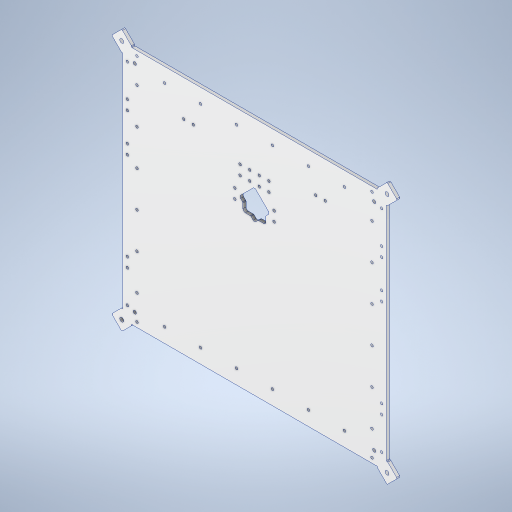
# Autodesk Inventor part: Printer Base Plate RevII
Saved by Autodesk Inventor 2024 (Build 280153000, 153)
## iProperties
Created: 2024-10-26
Part Number: Printer Base Plate RevII
Material: Aluminum 6061
Document SubType Name: Modeling
Designer: Ishaan
Density: 2.7 g/cm^3
Appearance: Aluminum - Flat
Author: Ishaan
Autodesk Inventor part; units mm, degrees
ref_plane "YZ Plane" through (0, 0, 0) normal (1, 0, 0) x (0, 1, 0)
ref_plane "XZ Plane" through (0, 0, 0) normal (0, 1, 0) x (-1, 0, 0)
ref_plane "XY Plane" through (0, 0, 0) normal (0, 0, 1) x (1, 0, 0)
sketch "Sketch1" plane through (0, 0, 0) normal (0, 0, 1) x (1, 0, 0)
  line L0 (275, -250) -> (-275, -250)
  line L1 (-275, -250) -> (-275, 250)
  line L2 (-275, 250) -> (275, 250)
  line L3 (275, 250) -> (275, -250)
  line L4 (275, -250) -> (-275, 250) construction
  line L5 (-275, -250) -> (275, 250) construction
  point P0 (0, 0)
  dimension "d0" = 550
  dimension "d1" = 500
  constraints: 12 end point, 2 midpoint, 2 parallel, 1 horizontal, 1 perpendicular
  measures "d0" distance of L1.end L2.end
  measures "d1" distance of L0.end L1.end
extrude "Extrusion1" add sketch "Sketch1" against normal blind 6.35
sketch "Sketch2" plane through (0, 0, 0) normal (0, 0, 1) x (1, 0, 0)
  line L0 (-235, 210) -> (-275, 210) construction
  line L1 (-275, 210) -> (-275, 250) construction
  line L2 (-275, 250) -> (-235, 250) construction
  line L3 (-235, 250) -> (-235, 210) construction
  line L4 (-235, 210) -> (-275, 250) construction
  line L5 (-275, 210) -> (-235, 250) construction
  line L6 (275, 210) -> (235, 210) construction
  line L7 (235, 210) -> (235, 250) construction
  line L8 (235, 250) -> (275, 250) construction
  line L9 (275, 250) -> (275, 210) construction
  line L10 (275, 210) -> (235, 250) construction
  line L11 (235, 210) -> (275, 250) construction
  line L12 (40, 122) -> (-40, 122) construction
  line L13 (-40, 122) -> (-40, 162) construction
  line L14 (-40, 162) -> (40, 162) construction
  line L15 (40, 162) -> (40, 122) construction
  line L16 (40, 122) -> (-40, 162) construction
  line L17 (-40, 122) -> (40, 162) construction
  line L18 (-235, -250) -> (-275, -250) construction
  line L19 (-275, -250) -> (-275, -210) construction
  line L20 (-275, -210) -> (-235, -210) construction
  line L21 (-235, -210) -> (-235, -250) construction
  line L22 (-235, -250) -> (-275, -210) construction
  line L23 (-275, -250) -> (-235, -210) construction
  line L24 (-275, 250) -> (-275, -250) construction
  line L25 (-275, -250) -> (275, -250) construction
  line L26 (275, -250) -> (235, -250) construction
  line L27 (235, -250) -> (235, -210) construction
  line L28 (235, -210) -> (275, -210) construction
  line L29 (275, -210) -> (275, -250) construction
  line L30 (275, -250) -> (235, -210) construction
  line L31 (235, -250) -> (275, -210) construction
  line L32 (275, -250) -> (275, 250) construction
  line L33 (-255, 122) -> (-275, 122) construction
  line L34 (-275, 122) -> (-275, 162) construction
  line L35 (-275, 162) -> (-255, 162) construction
  line L36 (-255, 162) -> (-255, 122) construction
  line L37 (-255, 122) -> (-275, 162) construction
  line L38 (-275, 122) -> (-255, 162) construction
  line L39 (275, 122) -> (255, 122) construction
  line L40 (255, 122) -> (255, 162) construction
  line L41 (255, 162) -> (275, 162) construction
  line L42 (275, 162) -> (275, 122) construction
  line L43 (275, 122) -> (255, 162) construction
  line L44 (255, 122) -> (275, 162) construction
  line L45 (-117.5, 165) -> (-157.5, 165) construction
  line L46 (-157.5, 165) -> (-157.5, 185) construction
  line L47 (-157.5, 185) -> (-117.5, 185) construction
  line L48 (-117.5, 185) -> (-117.5, 165) construction
  line L49 (-117.5, 165) -> (-157.5, 185) construction
  line L50 (-157.5, 165) -> (-117.5, 185) construction
  line L51 (157.5, 165) -> (117.5, 165) construction
  line L52 (117.5, 165) -> (117.5, 185) construction
  line L53 (117.5, 185) -> (157.5, 185) construction
  line L54 (157.5, 185) -> (157.5, 165) construction
  line L55 (157.5, 165) -> (117.5, 185) construction
  line L56 (117.5, 165) -> (157.5, 185) construction
  line L57 (-137.5, 175) -> (137.5, 175) construction
  line L58 (-255, -162) -> (-275, -162) construction
  line L59 (-275, -162) -> (-275, -122) construction
  line L60 (-275, -122) -> (-255, -122) construction
  line L61 (-255, -122) -> (-255, -162) construction
  line L62 (-255, -162) -> (-275, -122) construction
  line L63 (-275, -162) -> (-255, -122) construction
  line L64 (-255, 42) -> (-275, 42) construction
  line L65 (-275, 42) -> (-275, 82) construction
  line L66 (-275, 82) -> (-255, 82) construction
  line L67 (-255, 82) -> (-255, 42) construction
  line L68 (-255, 42) -> (-275, 82) construction
  line L69 (-275, 42) -> (-255, 82) construction
  line L70 (275, 42) -> (255, 42) construction
  line L71 (255, 42) -> (255, 82) construction
  line L72 (255, 82) -> (275, 82) construction
  line L73 (275, 82) -> (275, 42) construction
  line L74 (275, 42) -> (255, 82) construction
  line L75 (255, 42) -> (275, 82) construction
  line L76 (275, -162) -> (255, -162) construction
  line L77 (255, -162) -> (255, -122) construction
  line L78 (255, -122) -> (275, -122) construction
  line L79 (275, -122) -> (275, -162) construction
  line L80 (275, -162) -> (255, -122) construction
  line L81 (255, -162) -> (275, -122) construction
  line L82 (-275, 220) -> (-235, 220) construction
  line L83 (-275, -250) -> (-275, 250) construction
  line L84 (-275, 132) -> (-255, 132) construction
  line L85 (-275, -220) -> (-235, -220) construction
  line L86 (-275, -132) -> (-255, -132) construction
  line L87 (-255, 42) -> (-255, -122) construction
  line L88 (-255, -40) -> (0, -40) construction
  line L89 (0, 122) -> (0, -250) construction
  line L90 (-245, 220) -> (-265, 220) construction
  line L91 (-265, 220) -> (-265, 240) construction
  line L92 (-265, 240) -> (-245, 240) construction
  line L93 (-245, 240) -> (-245, 220) construction
  line L94 (-245, 220) -> (-265, 240) construction
  line L95 (-265, 220) -> (-245, 240) construction
  line L96 (265, 220) -> (245, 220) construction
  line L97 (245, 220) -> (245, 240) construction
  line L98 (245, 240) -> (265, 240) construction
  line L99 (265, 240) -> (265, 220) construction
  line L100 (265, 220) -> (245, 240) construction
  line L101 (245, 220) -> (265, 240) construction
  line L102 (265, 152) -> (265, 132) construction
  line L103 (265, 72) -> (265, 52) construction
  line L104 (265, -132) -> (265, -152) construction
  line L105 (-265, 152) -> (-265, 132) construction
  line L106 (-265, 72) -> (-265, 52) construction
  line L107 (-265, -132) -> (-265, -152) construction
  line L108 (-147.5, 175) -> (-127.5, 175) construction
  line L109 (127.5, 175) -> (147.5, 175) construction
  line L110 (265, -240) -> (245, -240) construction
  line L111 (245, -240) -> (245, -220) construction
  line L112 (245, -220) -> (265, -220) construction
  line L113 (265, -220) -> (265, -240) construction
  line L114 (265, -240) -> (245, -220) construction
  line L115 (245, -240) -> (265, -220) construction
  line L116 (-245, -240) -> (-265, -240) construction
  line L117 (-265, -240) -> (-265, -220) construction
  line L118 (-265, -220) -> (-245, -220) construction
  line L119 (-245, -220) -> (-245, -240) construction
  line L120 (-245, -240) -> (-265, -220) construction
  line L121 (-265, -240) -> (-245, -220) construction
  line L122 (10, 132) -> (-10, 132) construction
  line L123 (-10, 132) -> (-10, 152) construction
  line L124 (-10, 152) -> (10, 152) construction
  line L125 (10, 152) -> (10, 132) construction
  line L126 (10, 132) -> (-10, 152) construction
  line L127 (-10, 132) -> (10, 152) construction
  line L128 (30, 132) -> (-30, 132) construction
  line L129 (-30, 132) -> (-30, 152) construction
  line L130 (-30, 152) -> (30, 152) construction
  line L131 (30, 152) -> (30, 132) construction
  line L132 (30, 132) -> (-30, 152) construction
  line L133 (-30, 132) -> (30, 152) construction
  point P0 (0, 0)
  point P1 (-255, 230)
  point P2 (255, 230)
  point P3 (0, 142)
  point P4 (-255, -230)
  point P5 (255, -230)
  point P6 (0, 175)
  point P7 (265, 142)
  point P8 (265, 62)
  point P9 (265, -142)
  point P10 (-265, -142)
  point P11 (-265, 62)
  point P12 (-265, 142)
  point P13 (0, 142)
  dimension "d4" = 40
  dimension "d5" = 40
  dimension "d6" = 40
  dimension "d7" = 40
  dimension "d8" = 80
  dimension "d9" = 40
  dimension "d10" = 40
  dimension "d11" = 40
  dimension "d13" = 40
  dimension "d14" = 40
  dimension "d15" = 20
  dimension "d16" = 40
  dimension "d17" = 20
  dimension "d18" = 40
  dimension "d19" = 40
  dimension "d20" = 20
  dimension "d21" = 40
  dimension "d22" = 20
  dimension "d23" = 3
  dimension "d24" = 275
  dimension "d25" = 20
  dimension "d26" = 40
  dimension "d27" = 20
  dimension "d28" = 40
  dimension "d29" = 20
  dimension "d30" = 40
  dimension "d31" = 20
  dimension "d32" = 40
  dimension "d33" = 392
  dimension "d35" = 10
  dimension "d36" = 10
  dimension "d37" = 88
  dimension "d40" = 88
  dimension "d42" = 48
  dimension "d44" = 164
  dimension "d49" = 10
  dimension "d51" = 162
  dimension "d52" = 20
  dimension "d53" = 20
  dimension "d54" = 20
  dimension "d55" = 20
  dimension "d56" = 20
  dimension "d57" = 20
  dimension "d58" = 20
  dimension "d59" = 20
  dimension "d60" = 20
  dimension "d61" = 20
  dimension "d62" = 20
  dimension "d63" = 20
  dimension "d64" = 20
  dimension "d65" = 20
  dimension "d66" = 20
  dimension "d67" = 20
  dimension "d68" = 20
  dimension "d69" = 20
  dimension "d70" = 60
  dimension "d71" = 20
  dimension "d79" = 10
  dimension "d87" = 80
  constraints: 260 end point, 52 midpoint, 38 parallel, 33 coincident, 23 perpendicular, 22 horizontal, 13 collinear, 6 vertical, 5 point on line, 2 horizontal alignment, 2 vertical alignment, 4 other
  measures "d4" distance of L1.end L2.end
  measures "d5" distance of L0.end L1.end
  measures "d6" distance of L7.end L8.end
  measures "d7" distance of L6.end L7.end
  measures "d8" distance of L13.end L14.end
  measures "d9" distance of L12.end L13.end
  measures "d10" distance of L19.end L20.end
  measures "d11" distance of L18.end L19.end
  measures "d13" distance of L27.end L28.end
  measures "d14" distance of L26.end L27.end
  measures "d15" distance of L34.end L35.end
  measures "d16" distance of L33.end L34.end
  measures "d17" distance of L40.end L41.end
  measures "d18" distance of L39.end L40.end
  measures "d19" distance of L46.end L47.end
  measures "d20" distance of L45.end L46.end
  measures "d21" distance of L52.end L53.end
  measures "d22" distance of L51.end L52.end
  measures "d23" distance between parallel lines of L14 L45
  measures "d24" distance of L57.start L57.end
  measures "d25" distance of L59.end L60.end
  measures "d26" distance of L58.end L59.end
  measures "d27" distance of L65.end L66.end
  measures "d28" distance of L64.end L65.end
  measures "d29" distance of L71.end L72.end
  measures "d30" distance of L70.end L71.end
  measures "d31" distance of L77.end L78.end
  measures "d32" distance of L76.end L77.end
  measures "d33" distance from line of L25 point (0, 142)
  measures "d35" distance between parallel lines of L82 L0
  measures "d36" distance between parallel lines of L33 L84
  measures "d37" distance between parallel lines of L82 L84
  measures "d40" distance between parallel lines of L86 L85
  measures "d42" distance between parallel lines of L20 L58
  measures "d44" distance between parallel lines of L60 L64
  measures "d49" distance between parallel lines of L60 L86
  measures "d51" distance between parallel lines of L12 L88
  measures "d52" distance of L91.end L92.end
  measures "d53" distance of L90.end L91.end
  measures "d54" distance of L97.end L98.end
  measures "d55" distance of L96.end L97.end
  measures "d56" distance of L102.start L102.end
  measures "d57" distance of L103.start L103.end
  measures "d58" distance of L104.start L104.end
  measures "d59" distance of L105.start L105.end
  measures "d60" distance of L106.start L106.end
  measures "d61" distance of L107.start L107.end
  measures "d62" distance of L108.start L108.end
  measures "d63" distance of L109.start L109.end
  measures "d64" distance of L111.end L112.end
  measures "d65" distance of L110.end L111.end
  measures "d66" distance of L117.end L118.end
  measures "d67" distance of L116.end L117.end
  measures "d68" distance of L123.end L124.end
  measures "d69" distance of L122.end L123.end
  measures "d70" distance of L129.end L130.end
  measures "d71" distance of L128.end L129.end
  measures "d79" distance between parallel lines of L20 L85
  measures "d87" distance between parallel lines of L66 L35
hole "Hole1" at (-245, 240, 0) at (-265, 220, 0) at (245, 240, 0) at (265, 220, 0) at (265, 152, 0) at (265, 132, 0) at (265, 52, 0) at (265, 72, 0) at (265, -152, 0) at (265, -132, 0) at (-265, 132, 0) at (-265, 152, 0) at (-265, 52, 0) at (-265, 72, 0) at (-265, -152, 0) at (-265, -132, 0) at (-127.5, 175, 0) at (-147.5, 175, 0) at (147.5, 175, 0) at (127.5, 175, 0) at (-265, -220, 0) at (-245, -240, 0) at (245, -240, 0) at (265, -220, 0) at (-30, 152, 0) at (-30, 132, 0) at (-10, 132, 0) at (-10, 152, 0) at (10, 152, 0) at (10, 132, 0) at (30, 132, 0) at (30, 152, 0) direction (0, 0, -1) diameter 5.3 end through all
sketch "Sketch3" plane through (0, 0, 0) normal (0, 0, 1) x (1, 0, 0)
  line L0 (41, 84) -> (-41, 84) construction
  line L1 (-41, 84) -> (-41, 104) construction
  line L2 (-41, 104) -> (41, 104) construction
  line L3 (41, 104) -> (41, 84) construction
  line L4 (41, 84) -> (-41, 104) construction
  line L5 (-41, 84) -> (41, 104) construction
  line L6 (40, 122) -> (-40, 122) construction
  line L7 (-2.8284, 65.0086) -> (-28.9914, 91.1716)
  line L8 (-28.9914, 96.8284) -> (-2.8284, 122.9914)
  line L9 (2.8284, 122.9914) -> (28.9914, 96.8284)
  line L10 (28.9914, 91.1716) -> (2.8284, 65.0086)
  line L11 (0, 62.1802) -> (0, 125.8198) construction
  line L12 (-31.8198, 94) -> (31.8198, 94) construction
  arc A0 (2.8284, 122.9914) -> (-2.8284, 122.9914) centre (0, 120.163) ccw
  arc A1 (28.9914, 91.1716) -> (28.9914, 96.8284) centre (26.163, 94) ccw
  arc A2 (-2.8284, 65.0086) -> (2.8284, 65.0086) centre (0, 67.837) ccw
  arc A3 (-28.9914, 96.8284) -> (-28.9914, 91.1716) centre (-26.163, 94) ccw
  line L13 (19, 70) -> (-19, 70)
  line L14 (-24, 75) -> (-24, 118)
  line L15 (-24, 118) -> (24, 118)
  line L16 (24, 118) -> (24, 75)
  line L17 (24, 70) -> (-24, 118) construction
  line L18 (-24, 70) -> (24, 118) construction
  arc A4 (-24, 75) -> (-19, 70) centre (-19, 75) ccw
  arc A5 (19, 70) -> (24, 75) centre (19, 75) ccw
  point P0 (0, 0)
  point P1 (0, 94)
  point P2 (0, 122)
  point P3 (24, 86.1802)
  point P4 (7.8198, 70)
  point P5 (-7.8198, 70)
  point P6 (-24, 86.1802)
  dimension "d88" = 82
  dimension "d89" = 20
  dimension "d90" = 28
  dimension "d201" = 45
  dimension "d202" = 4
  dimension "d205" = 48
  dimension "d206" = 48
  dimension "d207" = 5
  constraints: 36 end point, 12 point on circle, 12 point on line, 12 tangent, 7 midpoint, 6 centre point, 6 parallel, 4 coincident, 4 equal radius, 4 perpendicular, 2 horizontal, 1 vertical, 1 vertical alignment
  measures "d88" distance of L1.end L2.end
  measures "d89" distance of L0.end L1.end
  measures "d90" distance from line of L6 point (0, 94)
  measures "d201" distance of L11.end L12.end
  measures "d202" radius of A0
  measures "d205" distance of L14.end L15.end
  measures "d206" distance of L18.start L14.end
  measures "d207" radius of A4
hole "Hole2" at (-41, 104, 0) at (-41, 84, 0) at (41, 104, 0) at (41, 84, 0) direction (0, 0, -1) diameter 5.3 end through all
extrude "Extrusion5" cut sketch "Sketch3" against normal through all contours L7 L13 L10 A2 | L13 A4 L14 L7 | L7 L14 L8 L15 L9 L16 L10 L13 | L7 A3 L8 L14 | L10 L16 A5 L13 | L16 L9 A1 L10 | L8 A0 L9 L15
sketch "Sketch4" plane through (0, 0, 0) normal (0, 0, 1) x (1, 0, 0)
  circle A0 centre (41, 84) radius 2.65 projected
  circle A1 centre (41, 104) radius 2.65 projected
  circle A2 centre (-41, 84) radius 2.65 projected
  circle A3 centre (-41, 104) radius 2.65 projected
  circle A4 centre (30, 152) radius 2.65 projected
  circle A5 centre (30, 132) radius 2.65 projected
  circle A6 centre (10, 132) radius 2.65 projected
  circle A7 centre (10, 152) radius 2.65 projected
  circle A8 centre (-10, 152) radius 2.65 projected
  circle A9 centre (-10, 132) radius 2.65 projected
  circle A10 centre (-30, 132) radius 2.65 projected
  circle A11 centre (-30, 152) radius 2.65 projected
  circle A12 centre (265, -220) radius 2.65 projected
  circle A13 centre (245, -240) radius 2.65 projected
  circle A14 centre (-245, -240) radius 2.65 projected
  circle A15 centre (-265, -220) radius 2.65 projected
  circle A16 centre (127.5, 175) radius 2.65 projected
  circle A17 centre (147.5, 175) radius 2.65 projected
  circle A18 centre (-147.5, 175) radius 2.65 projected
  circle A19 centre (-127.5, 175) radius 2.65 projected
  circle A20 centre (-265, -132) radius 2.65 projected
  circle A21 centre (-265, -152) radius 2.65 projected
  circle A22 centre (-265, 72) radius 2.65 projected
  circle A23 centre (-265, 52) radius 2.65 projected
  circle A24 centre (-265, 152) radius 2.65 projected
  circle A25 centre (-265, 132) radius 2.65 projected
  circle A26 centre (265, -132) radius 2.65 projected
  circle A27 centre (265, -152) radius 2.65 projected
  circle A28 centre (265, 72) radius 2.65 projected
  circle A29 centre (265, 52) radius 2.65 projected
  circle A30 centre (265, 132) radius 2.65 projected
  circle A31 centre (265, 152) radius 2.65 projected
  circle A32 centre (265, 220) radius 2.65 projected
  circle A33 centre (245, 240) radius 2.65 projected
  circle A34 centre (-265, 220) radius 2.65 projected
  circle A35 centre (-245, 240) radius 2.65 projected
  line L0 (275, 250) -> (-275, 250) projected
  line L1 (-275, 250) -> (-275, -250) projected
  line L2 (-275, -250) -> (275, -250) projected
  line L3 (275, -250) -> (275, 250) projected
  line L4 (-235, 228.5) -> (-255, 228.5) construction
  line L5 (-255, 228.5) -> (-255, 251.5) construction
  line L6 (-255, 251.5) -> (-235, 251.5) construction
  line L7 (-235, 251.5) -> (-235, 228.5) construction
  line L8 (-235, 228.5) -> (-255, 251.5) construction
  line L9 (-255, 228.5) -> (-235, 251.5) construction
  line L10 (-253.5, 210) -> (-276.5, 210) construction
  line L11 (-276.5, 210) -> (-276.5, 230) construction
  line L12 (-276.5, 230) -> (-253.5, 230) construction
  line L13 (-253.5, 230) -> (-253.5, 210) construction
  line L14 (-253.5, 210) -> (-276.5, 230) construction
  line L15 (-276.5, 210) -> (-253.5, 230) construction
  line L16 (-277.9142, 231.701) -> (-296.299, 250.0858)
  line L17 (-296.299, 252.9142) -> (-277.9142, 271.299)
  line L18 (-275.0858, 271.299) -> (-256.701, 252.9142)
  line L19 (-256.701, 250.0858) -> (-275.0858, 231.701)
  line L20 (-276.5, 230.2868) -> (-276.5, 272.7132) construction
  line L21 (-297.7132, 251.5) -> (-255.2868, 251.5) construction
  line L22 (275, 250) -> (-275, 250) projected
  line L23 (276.5, -251.5) -> (-276.5, -251.5) construction
  line L24 (-276.5, -251.5) -> (-276.5, 251.5) construction
  line L25 (-276.5, 251.5) -> (276.5, 251.5) construction
  line L26 (276.5, 251.5) -> (276.5, -251.5) construction
  line L27 (276.5, -251.5) -> (-276.5, 251.5) construction
  line L28 (-276.5, -251.5) -> (276.5, 251.5) construction
  line L29 (275, -250) -> (275, 250) projected
  arc A36 (-275.0858, 271.299) -> (-277.9142, 271.299) centre (-276.5, 269.8848) ccw
  arc A37 (-256.701, 250.0858) -> (-256.701, 252.9142) centre (-258.1152, 251.5) ccw
  arc A38 (-277.9142, 231.701) -> (-275.0858, 231.701) centre (-276.5, 233.1152) ccw
  arc A39 (-296.299, 252.9142) -> (-296.299, 250.0858) centre (-294.8848, 251.5) ccw
  circle A40 centre (-255.1572, 251) radius 1
  circle A41 centre (-276, 230.1572) radius 1
  line L30 (-275, 250) -> (-275, -250) projected
  point P0 (0, 0)
  point P1 (-275, 231.7868)
  point P2 (-256.7868, 250)
  point P3 (-255.1572, 250)
  point P4 (-256.1432, 251.1667)
  point P5 (-276.1667, 231.1432)
  point P6 (-275, 230.1572)
  dimension "d156" = 20
  dimension "d157" = 23
  dimension "d158" = 23
  dimension "d159" = 20
  dimension "d160" = 30
  dimension "d161" = 30
  dimension "d162" = 2
  dimension "d163" = 2
  constraints: 48 end point, 12 tangent, 9 point on line, 8 midpoint, 8 parallel, 8 point on circle, 6 centre point, 4 equal radius, 4 perpendicular, 3 horizontal, 1 coincident, 1 collinear, 1 vertical
  measures "d156" distance of L5.end L6.end
  measures "d157" distance of L4.end L5.end
  measures "d158" distance of L11.end L12.end
  measures "d159" distance of L10.end L11.end
  measures "d160" distance of L21.start L20.end
  measures "d161" distance of L20.end L21.end
  measures "d162" radius of A36
  measures "d163" diameter of A40
extrude "Extrusion2" add sketch "Sketch4" against normal up to surface (6.35 mm away) contours L0 L19 A37 A40 | L0 L1 L19 A38 L16 A39 L17 A36 L18 A37 | L1 A41 A38 L19
fillet "Fillet2" radius 2 4 edges at (-7.8198, 70, -3.175) (-24, 86.1802, -3.175) (7.8198, 70, -3.175) (24, 86.1802, -3.175)
hole "Hole6" at (-276.5, 251.5, 0) direction (0, 0, -1) diameter 8.3 end through all
mirror "Mirror1" about plane through (0, 0, 0) normal (1, 0, 0) of "Extrusion2", "Hole6"
mirror "Mirror2" about plane through (0, 0, 0) normal (0, 1, 0) of "Extrusion2", "Hole6", "Mirror1"
sketch "Sketch7" plane through (0, 0, 0) normal (0, 0, 1) x (1, 0, 0)
  line L0 (245, -220) -> (-245, -220) construction
  line L1 (-245, -220) -> (-245, 220) construction
  line L2 (-245, 220) -> (245, 220) construction
  line L3 (245, 220) -> (245, -220) construction
  line L4 (245, -220) -> (-245, 220) construction
  line L5 (-245, -220) -> (245, 220) construction
  line L6 (-37.5, 220) -> (37.5, 220) construction
  point P0 (0, 0)
  point P1 (-187.5, 220)
  point P2 (-112.5, 220)
  point P3 (112.5, 220)
  point P4 (187.5, 220)
  point P5 (0, 220)
  dimension "d118" = 490
  dimension "d119" = 440
  dimension "d194" = 75
  dimension "d200" = 375
  constraints: 14 end point, 4 midpoint, 3 horizontal, 2 parallel, 1 perpendicular, 5 other
  measures "d118" distance of L1.end L2.end
  measures "d119" distance of L0.end L1.end
  measures "d194" distance of point (-187.5, 220) point (-112.5, 220)
  measures "d200" distance of point (187.5, 220) point (-187.5, 220)
hole "Hole4" at (187.5, 220, 0) at (112.5, 220, 0) at (37.5, 220, 0) at (-37.5, 220, 0) at (-112.5, 220, 0) at (-187.5, 220, 0) direction (0, 0, -1) diameter 5.3 end through all
mirror "Mirror3" about plane through (0, 0, 0) normal (0, 1, 0) of "Hole4"
sketch "Sketch9" plane through (0, 0, 0) normal (0, 0, 1) x (1, 0, 0)
  line L0 (-245, -220) -> (-245, 220) construction
  line L1 (-245, -37.5) -> (-245, 37.5) construction
  point P0 (0, 0)
  point P1 (-245, 187.5)
  point P2 (-245, 112.5)
  point P3 (-245, -112.5)
  point P4 (-245, -187.5)
  point P5 (-245, 0)
  dimension "d175" = 440
  dimension "d178" = 75
  dimension "d183" = 375
  constraints: 2 end point, 2 midpoint, 2 vertical, 5 other
  measures "d175" distance of L0.start L0.end
  measures "d178" distance of point (-245, 187.5) point (-245, 112.5)
  measures "d183" distance of point (-245, 187.5) point (-245, -187.5)
hole "Hole7" at (-245, 187.5, 0) at (-245, 112.5, 0) at (-245, 37.5, 0) at (-245, -37.5, 0) at (-245, -112.5, 0) at (-245, -187.5, 0) direction (0, 0, -1) diameter 5.3 end through all
mirror "Mirror4" about plane through (0, 0, 0) normal (1, 0, 0) of "Hole7"
sketch "Sketch8" plane through (0, 0, 0) normal (0, 0, 1) x (1, 0, 0)
  line L0 (-249.5, 224.5) -> (249.5, 224.5) construction
  line L1 (249.5, 224.5) -> (249.5, -224.5) construction
  line L2 (249.5, -224.5) -> (-249.5, -224.5) construction
  line L3 (-249.5, -224.5) -> (-249.5, 224.5) construction
  line L4 (-249.5, 224.5) -> (249.5, -224.5) construction
  line L5 (249.5, 224.5) -> (-249.5, -224.5) construction
  circle A0 centre (249.5, -224.5) radius 6.5 construction
  point P0 (0, 0)
  dimension "d138" = 499
  dimension "d139" = 449
  dimension "d140" = 13
  constraints: 12 end point, 5 coincident, 2 midpoint, 2 parallel, 1 centre point, 1 horizontal, 1 perpendicular
  measures "d138" distance of L1.end L2.end
  measures "d139" distance of L0.end L1.end
  measures "d140" diameter of A0
hole "Hole5" at (-249.5, 224.5, 0) at (249.5, 224.5, 0) at (249.5, -224.5, 0) at (-249.5, -224.5, 0) direction (0, 0, -1) diameter 6.647 end through all thread size "M8x1.25" class "6H" standard "ANSI Metric M Profile"
equation "\"d40\" = d37"
body "Solid1"
